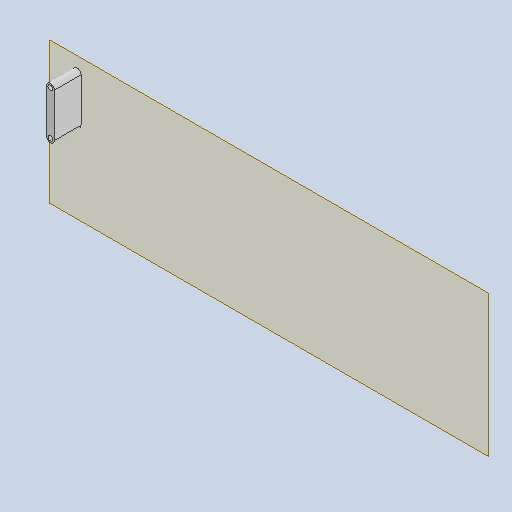
# Autodesk Inventor part: plate_washer_1
Saved by Autodesk Inventor 2024 (Build 280153000, 153)
## iProperties
Created: 2026-02-04
Part Number: plate_washer_1
Material: Generic
Document SubType Name: Modeling
Designer: SEMEN
Density: 1 g/cm^3
Appearance: Default
Author: SEMEN
Autodesk Inventor part; units mm, degrees
ref_plane "YZ Plane" through (0, 0, 0) normal (1, 0, 0) x (0, 1, 0)
ref_plane "XZ Plane" through (0, 0, 0) normal (0, 1, 0) x (-1, 0, 0)
ref_plane "XY Plane" through (0, 0, 0) normal (0, 0, 1) x (1, 0, 0)
ref_plane "Work Plane1" through (0, 0, 0) normal (0, 0, 1) x (1, 0, 0)
sketch "Sketch1" plane through (0, 0, 0) normal (0, 0, 1) x (1, 0, 0)
  circle A0 centre (-26, -14) radius 1.7 projected
  circle A1 centre (-26, 15.5) radius 1.7 projected
  arc A2 (-28.7, -14) -> (-23.3, -14) centre (-26, -14) ccw
  arc A3 (-23.3, 15.5) -> (-28.7, 15.5) centre (-26, 15.5) ccw
  line L0 (-28.7, -14) -> (-28.7, 15.5)
  line L1 (-26, -14) -> (-28.7, -14) construction
  line L2 (-203.2094, -16) -> (37.4788, -16) construction
  line L3 (-27.8138, -16) -> (-106.7251, -16)
  line L4 (-23.3, -14) -> (-23.3, 15.5)
  point P0 (0, 0)
  dimension "d12" = 16
  dimension "d13" = 1
  constraints: 10 end point, 6 point on circle, 2 centre point, 2 horizontal, 2 point on line, 2 tangent, 1 equal radius, 1 perpendicular
  measures "d12" distance from line of L2 point (0, 0)
  measures "d13" radial gap between concentric circles of A3 A1
extrude "Extrusion1" add sketch "Sketch1" along normal blind 18 contours A0 | A1 | L0 A3 L4 A2
hole "Hole1" at (-26, 15.5, 0) at (-26, -14, 0) direction (0, 0, 1) diameter 3.4 end through all clearance for "Countersunk Head GOST 12876-67" size "M3" standard "GOST"
body "Solid1"
